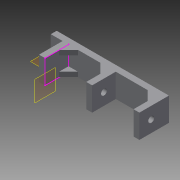
# Autodesk Inventor part: side
Saved by Autodesk Inventor 2013 (Build 170138000, 138)
## iProperties
Created: 2013-02-01
Part Number: side
Material: Generic
Document SubType Name: Modeling
Designer: Brad
Density: 1 g/cm^3
Author: Brad
Autodesk Inventor part; units mm, degrees
ref_plane "YZ Plane" through (0, 0, 0) normal (1, 0, 0) x (0, 1, 0)
ref_plane "XZ Plane" through (0, 0, 0) normal (0, 1, 0) x (-1, 0, 0)
ref_plane "XY Plane" through (0, 0, 0) normal (0, 0, 1) x (1, 0, 0)
sketch "Sketch1" plane through (0, 0, 0) normal (0, 0, 1) x (1, 0, 0)
  line L0 (-11.658, 3.4387) -> (-11.658, -21.9613)
  line L1 (-11.658, 3.4387) -> (108.992, 3.4387)
  line L2 (108.992, 3.4387) -> (108.992, -21.9613)
  line L3 (108.992, -21.9613) -> (-11.658, -21.9613)
  point P0 (0, 0)
  dimension "d0" = 25.4
  dimension "d1" = 120.65
  dimension "d2" = 25.4
  constraints: 8 end point, 2 perpendicular, 1 vertical
  measures "d0" distance of L0.start L0.end
  measures "d1" distance of L0.start L1.end
  measures "d2" distance of L1.end L2.end
extrude "Extrusion1" add sketch "Sketch1" along normal blind 6.35
ref_plane "Work Plane1" through (-11.658, -21.9613, 6.35) normal (0, 1, 0) x (1, 0, 0)
sketch "Sketch3" plane through (-11.658, -21.9613, 6.35) normal (0, 1, 0) x (1, 0, 0)
  line L0 (0, 0) -> (120.65, 0) projected
  line L1 (120.65, -25.4) -> (0, -25.4) projected
  line L2 (120.65, 0) -> (120.65, -25.4) projected
  line L3 (0, -25.4) -> (12.7, -25.4)
  line L4 (12.7, -25.4) -> (12.7, 0)
  line L5 (12.7, 0) -> (19.05, 0)
  line L6 (19.05, 0) -> (19.05, -25.4)
  line L7 (19.05, -25.4) -> (12.7, -25.4)
  line L8 (19.05, -25.4) -> (63.5, -25.4)
  line L9 (63.5, -25.4) -> (63.5, 0)
  line L10 (63.5, 0) -> (69.85, 0)
  line L11 (69.85, 0) -> (69.85, -25.4)
  line L12 (69.85, -25.4) -> (63.5, -25.4)
  line L13 (69.85, -25.4) -> (114.3, -25.4)
  line L14 (114.3, -25.4) -> (114.3, 0)
  line L15 (120.65, 0) -> (114.3, 0)
  line L16 (120.65, 0) -> (120.65, -25.4)
  line L17 (114.3, -25.4) -> (120.65, -25.4)
  point P0 (11.658, 6.35)
  dimension "d8" = 12.7
  dimension "d9" = 6.35
  dimension "d10" = 25.4
  dimension "d11" = 44.45
  dimension "d12" = 6.35
  dimension "d13" = 25.4
  dimension "d14" = 44.45
  constraints: 30 end point, 10 point on line, 5 perpendicular, 3 collinear
  measures "d8" distance of L1.end L3.end
  measures "d9" distance of L4.end L5.end
  measures "d10" distance of L5.end L6.end
  measures "d11" distance of L6.end L8.end
  measures "d12" distance of L9.end L10.end
  measures "d13" distance of L10.end L11.end
  measures "d14" distance of L11.end L13.end
extrude "Extrusion3" add sketch "Sketch3" along normal blind 25.4 contours L0 L6 L1 L4 | L0 L11 L1 L9 | L0 L2 L1 L14
ref_plane "Work Plane2" through (7.392, -21.9613, 31.75) normal (1, 0, 0) x (0, 0, -1)
sketch "Sketch4" plane through (7.392, -21.9613, 31.75) normal (1, 0, 0) x (0, 0, -1)
  line L0 (25.4, 0) -> (0, 0) projected
  line L1 (25.4, 25.4) -> (25.4, 0) projected
  line L2 (0, 25.4) -> (25.4, 25.4) projected
  line L3 (0, 0) -> (0, 25.4) projected
  point P0 (31.75, 21.9613)
sketch "Sketch5" plane through (108.992, -21.9613, 0) normal (1, 0, 0) x (0, 0, -1)
  line L0 (-31.75, 0) -> (-31.75, 31.75) projected
  line L1 (-31.75, 31.75) -> (-31.75, 12.7)
  line L2 (-31.75, 12.7) -> (-19.05, 12.7)
  circle A0 centre (-19.05, 12.7) radius 3.175
  point P0 (0, 21.9613)
  dimension "d17" = 19.05
  dimension "d18" = 12.7
  dimension "d19" = 6.35
  constraints: 4 end point, 1 centre point, 1 coincident, 1 perpendicular, 1 point on line
  measures "d17" distance of L0.end L1.end
  measures "d18" distance of L1.end L2.end
  measures "d19" diameter of A0
extrude "Extrusion4" cut sketch "Sketch5" against normal blind 76.2
sketch "Sketch6" plane through (-11.658, -21.9613, 0) normal (0, -1, 0) x (1, 0, 0)
  line L0 (114.3, 6.35) -> (114.3, 31.75) projected
  line L1 (69.85, 6.35) -> (114.3, 6.35) projected
  line L2 (63.5, 6.35) -> (63.5, 31.75) projected
  line L3 (19.05, 6.35) -> (63.5, 6.35) projected
  line L4 (19.05, 31.75) -> (19.05, 6.35) projected
  line L5 (19.05, 6.35) -> (19.05, 16.51)
  line L6 (19.05, 6.35) -> (29.21, 6.35)
  line L7 (29.21, 6.35) -> (19.05, 16.51)
  line L8 (63.5, 6.35) -> (53.34, 6.35)
  line L9 (53.34, 6.35) -> (63.5, 16.51)
  line L10 (63.5, 6.35) -> (63.5, 16.51)
  line L11 (114.3, 6.35) -> (104.14, 6.35)
  line L12 (104.14, 6.35) -> (114.3, 16.51)
  line L13 (114.3, 6.35) -> (114.3, 16.51)
  point P0 (11.658, 0)
  dimension "d22" = 10.16
  dimension "d23" = 10.16
  dimension "d24" = 10.16
  dimension "d25" = 10.16
  constraints: 18 end point, 6 point on line, 3 perpendicular, 1 parallel
  measures "d22" distance of L3.start L5.end
  measures "d23" distance of L3.start L6.end
  measures "d24" distance of L2.start L8.end
  measures "d25" distance of L0.start L11.end
extrude "Extrusion5" add sketch "Sketch6" against normal blind 5.08
sketch "Sketch7" plane through (-11.658, 3.4387, 0) normal (0, 1, 0) x (1, 0, 0)
  line L0 (19.05, -31.75) -> (19.05, -6.35) projected
  line L1 (63.5, -6.35) -> (19.05, -6.35) projected
  line L2 (63.5, -6.35) -> (63.5, -31.75) projected
  line L3 (19.05, -6.35) -> (19.05, -16.51)
  line L4 (19.05, -6.35) -> (29.21, -6.35)
  line L5 (29.21, -6.35) -> (19.05, -16.51)
  line L6 (63.5, -6.35) -> (53.34, -6.35)
  line L7 (53.34, -6.35) -> (63.5, -16.51)
  line L8 (63.5, -6.35) -> (63.5, -16.51)
  line L9 (114.3, -6.35) -> (104.14, -6.35)
  line L10 (104.14, -6.35) -> (114.3, -16.51)
  line L11 (114.3, -6.35) -> (114.3, -16.51)
  point P0 (11.658, 0)
  dimension "d28" = 10.16
  dimension "d29" = 10.16
  dimension "d30" = 10.16
  dimension "d31" = 10.16
  constraints: 18 end point, 4 point on line, 1 collinear, 1 perpendicular
  measures "d28" distance of L0.end L3.end
  measures "d29" distance of L0.end L4.end
  measures "d30" distance of L1.start L6.end
  measures "d31" distance of L11.start L10.start
extrude "Extrusion6" add sketch "Sketch7" against normal blind 5.08
body "Solid1"
